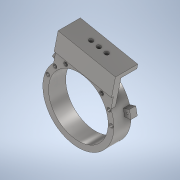
# Autodesk Inventor part: 02
Saved by Autodesk Inventor 2021 (Build 250183000, 183)
## iProperties
Created: 2021-01-15
Part Number: 02
Material: Edelstahl
Document SubType Name: Modeling
Designer: Daniel Dux
Density: 8 g/cm^3
Appearance: Halbpoliert
Mass: 1022.9 g
Surface Area: 385.122 cm^2
Volume: 127.862 cm^3
d117: 94,000 mm
d118: 112,000 mm
d119: 104,000 mm
d120: 5,000 mm
d121: 7,000 mm
d122: 94,000 mm
d123: 5,000 mm
d124: 10,000 mm
d125: 112,000 mm
d208: 98,000 mm
d209: 112,000 mm
d210: 104,000 mm
d211: 5,000 mm
d212: 7,000 mm
d213: 98,000 mm
d214: 5,000 mm
d215: 10,000 mm
d216: 112,000 mm
d217: 20,000 mm
d236: 94,000 mm
d237: 112,000 mm
d238: 104,000 mm
d239: 6,000 mm
d240: 7,000 mm
d241: 98,000 mm
d242: 8,000 mm
d243: 10,000 mm
Author: Daniel Dux
Title: Oberer Mount
Autodesk Inventor part; units mm, degrees
sketch "Skizze1" plane through (0, 0, 0) normal (0, 0, 1) x (1, 0, 0)
  circle A0 centre (0, 0) radius 47
  circle A1 centre (0, 0) radius 56
  circle A2 centre (0, 0) radius 51.5
  circle A3 centre (-28.6119, 42.8207) radius 6
  circle A4 centre (-42.8207, 28.6119) radius 6
  circle A5 centre (42.8207, 28.6119) radius 6
  circle A6 centre (50.5104, 10.0472) radius 6
  circle A7 centre (-10.0472, -50.5104) radius 6
  circle A8 centre (-28.6119, 42.8207) radius 5
  circle A9 centre (-42.8207, 28.6119) radius 5
  circle A10 centre (-10.0472, -50.5104) radius 5
  circle A11 centre (50.5104, 10.0472) radius 5
  circle A12 centre (42.8207, 28.6119) radius 5
  line L0 (0, 0) -> (-25.4753, 49.8699)
  line L1 (0, 0) -> (-26.4443, 49.3629)
  line L2 (0, 0) -> (-36.3248, 42.6205)
  line L3 (0, 0) -> (-35.4856, 43.3218)
  line L4 (0, 0) -> (-42.6205, 36.3248)
  line L5 (0, 0) -> (-49.3629, 26.4443)
  line L6 (0, 0) -> (-49.8699, 25.4753)
  line L7 (0, 0) -> (-43.3218, 35.4856)
  line L8 (0, 0) -> (-16.2059, -53.6038)
  line L9 (0, 0) -> (-17.2496, -53.2771)
  line L10 (0, 0) -> (-5.541, -55.7252)
  line L11 (0, 0) -> (-4.4517, -55.8228)
  line L12 (0, 0) -> (43.3218, 35.4856)
  line L13 (0, 0) -> (42.6205, 36.3248)
  line L14 (0, 0) -> (49.3629, 26.4443)
  line L15 (0, 0) -> (49.8699, 25.4753)
  line L16 (0, 0) -> (53.6038, 16.2059)
  line L17 (0, 0) -> (53.2771, 17.2496)
  line L18 (0, 0) -> (55.7252, 5.541)
  line L19 (0, 0) -> (55.8228, 4.4517)
  line L20 (0, 0) -> (-54.924, 10.9251)
  line L21 (0, 0) -> (54.924, -10.9251)
  line L22 (0, 0) -> (10.0472, 50.5104)
  point P0 (0, 51.5)
  point P1 (-10.0472, 50.5104)
  point P2 (-19.7082, 47.5798)
  point P3 (-36.416, 36.416)
  point P4 (-47.5798, 19.7082)
  point P5 (-50.5104, 10.0472)
  point P6 (-51.5, 0)
  point P7 (-50.5104, -10.0472)
  point P8 (-47.5798, -19.7082)
  point P9 (-42.8207, -28.6119)
  point P10 (-36.416, -36.416)
  point P11 (-28.6119, -42.8207)
  point P12 (-19.7082, -47.5798)
  point P13 (0, -51.5)
  point P14 (10.0472, -50.5104)
  point P15 (19.7082, -47.5798)
  point P16 (28.6119, -42.8207)
  point P17 (36.416, -36.416)
  point P18 (42.8207, -28.6119)
  point P19 (47.5798, -19.7082)
  point P20 (50.5104, -10.0472)
  point P21 (51.5, 0)
  point P22 (47.5798, 19.7082)
  point P23 (36.416, 36.416)
  point P24 (28.6119, 42.8207)
  point P25 (19.7082, 47.5798)
  point P26 (-41.8551, 21.3811)
  point P27 (-41.4296, 22.1944)
  point P28 (-36.3593, 29.7825)
  point P29 (-35.7708, 30.4869)
  point P30 (-30.3782, 37.0866)
  point P31 (-30.4869, 35.7708)
  point P32 (-29.1766, 36.8473)
  point P33 (-22.6383, 42.2582)
  point P34 (-22.8771, 41.0565)
  point P35 (-21.3811, 41.8551)
  point P36 (-14.4773, -44.7147)
  point P37 (-13.6014, -44.9889)
  point P38 (-3.7363, -46.8513)
  point P39 (-4.6505, -46.7694)
  point P40 (46.7694, 4.6505)
  point P41 (46.8513, 3.7363)
  point P42 (44.7147, 14.4773)
  point P43 (44.9889, 13.6014)
  point P44 (41.4296, 22.1944)
  point P45 (41.8551, 21.3811)
  point P46 (35.7708, 30.4869)
  point P47 (36.3593, 29.7825)
  dimension "d1" = 112
  dimension "d2" = 103
  dimension "d0" = 94
  dimension "d5" = 360
  dimension "d7" = 12
  dimension "d8" = 12
  dimension "d9" = 12
  dimension "d10" = 12
  dimension "d11" = 12
  dimension "d12" = 10
  dimension "d13" = 10
  dimension "d14" = 10
  dimension "d15" = 10
  dimension "d16" = 10
  constraints: 12 coincident, 11 centre point, 1 end point, 128 other
  measures "d0" diameter of A0
  measures "d7" diameter of A3
  measures "d8" diameter of A4
  measures "d9" diameter of A5
  measures "d10" diameter of A6
  measures "d11" diameter of A7
  measures "d12" diameter of A8
  measures "d13" diameter of A9
  measures "d14" diameter of A10
  measures "d15" diameter of A11
  measures "d16" diameter of A12
ref_plane "Arbeitsebene1" through (0, 0, 10) normal (0, 0, 1) x (1, 0, 0)
sketch "Skizze2" plane through (0, 0, 10) normal (0, 0, 1) x (1, 0, 0)
  circle A0 centre (0, 0) radius 47
  circle A1 centre (0, 0) radius 56
  arc A2 (-42.7016, 36.2295) -> (-43.3876, 35.405) centre (0, 0) ccw projected
  line L0 (0, 0) -> (-25.5867, 49.8129)
  arc A3 (55.8127, 4.5765) -> (55.7148, 5.6445) centre (0, 0) ccw projected
  line L1 (-22.3883, 43.5863) -> (-25.5867, 49.8129) projected
  circle A4 centre (0, 0) radius 47
  circle A5 centre (0, 0) radius 56
  circle A6 centre (0, 0) radius 52.5
  line L2 (0, 0) -> (-25.5867, 49.8129)
  point P0 (-21.4745, 41.8072)
  point P1 (0, 52.5)
  point P2 (-10.2422, 51.4912)
  point P3 (-20.0909, 48.5037)
  point P4 (-29.1674, 43.6522)
  point P5 (-37.1231, 37.1231)
  point P6 (-43.6522, 29.1674)
  point P7 (-48.5037, 20.0909)
  point P8 (-51.4912, 10.2422)
  point P9 (-52.5, 0)
  point P10 (-51.4912, -10.2422)
  point P11 (-48.5037, -20.0909)
  point P12 (-43.6522, -29.1674)
  point P13 (-37.1231, -37.1231)
  point P14 (-29.1674, -43.6522)
  point P15 (-20.0909, -48.5037)
  point P16 (-10.2422, -51.4912)
  point P17 (0, -52.5)
  point P18 (10.2422, -51.4912)
  point P19 (20.0909, -48.5037)
  point P20 (29.1674, -43.6522)
  point P21 (37.1231, -37.1231)
  point P22 (43.6522, -29.1674)
  point P23 (48.5037, -20.0909)
  point P24 (51.4912, -10.2422)
  point P25 (52.5, 0)
  point P26 (51.4912, 10.2422)
  point P27 (48.5037, 20.0909)
  point P28 (43.6522, 29.1674)
  point P29 (37.1231, 37.1231)
  point P30 (29.1674, 43.6522)
  point P31 (20.0909, 48.5037)
  point P32 (10.2422, 51.4912)
  point P33 (-43.5863, 22.3883)
  point P34 (-43.1495, 23.219)
  point P35 (-37.9642, 30.9794)
  point P36 (-37.3639, 31.7008)
  point P37 (-30.9445, 37.9213)
  point P38 (-31.7008, 37.3639)
  point P39 (-31.0074, 37.9413)
  point P40 (-23.1928, 43.1008)
  point P41 (-23.1871, 43.1666)
  point P42 (-14.9892, -46.6511)
  point P43 (-14.093, -46.9296)
  point P44 (-4.0044, -48.8361)
  point P45 (-4.939, -48.7505)
  point P46 (48.7505, 4.939)
  point P47 (48.8361, 4.0044)
  point P48 (46.6511, 14.9892)
  point P49 (46.9296, 14.093)
  point P50 (43.1495, 23.219)
  point P51 (43.5863, 22.3883)
  point P52 (37.3639, 31.7008)
  point P53 (37.9642, 30.9794)
  dimension "d19" = 94
  dimension "d81" = 112
  dimension "d82" = 105
  dimension "d20" = 112
  dimension "d80" = 94
  dimension "d83" = 360
  constraints: 5 coincident, 4 end point, 2 centre point, 1 collinear, 1 vertical alignment, 40 other
  measures "d20" diameter of A1
  measures "d80" diameter of A4
extrude "Extrusion2" add sketch "Skizze2" along normal blind 10 contours A1 | A6
ref_plane "Arbeitsebene2" through (0, 0, 20) normal (0, 0, 1) x (1, 0, 0)
sketch "Skizze3" plane through (0, 0, 20) normal (0, 0, 1) x (1, 0, 0)
  circle A0 centre (0, 0) radius 47
  circle A1 centre (0, 0) radius 56
  dimension "d30" = 94
  dimension "d31" = 112
  constraints: 2 centre point, 2 coincident
  measures "d30" diameter of A0
  measures "d31" diameter of A1
extrude "Extrusion3" add sketch "Skizze3" along normal blind 10
ref_plane "Arbeitsebene3" through (0, 0, 30) normal (0, 0, 1) x (1, 0, 0)
sketch "Skizze4" plane through (0, 0, 30) normal (0, 0, 1) x (1, 0, 0)
  circle A0 centre (0, 0) radius 49 projected
  line L0 (-22.188, 43.8818) -> (37.2918, 32.0506)
  line L1 (37.2918, 32.0506) -> (44.6056, 68.8203)
  line L2 (44.6056, 68.8203) -> (-14.8741, 80.6514)
  line L3 (-14.8741, 80.6514) -> (-22.188, 43.8818)
  line L4 (44.6056, 68.8203) -> (37.2918, 32.0506)
  line L5 (37.2918, 32.0506) -> (52.7171, 28.9824)
  line L6 (48.4587, 7.5737) -> (60.031, 65.752)
  line L7 (60.031, 65.752) -> (44.6056, 68.8203)
  line L8 (-14.8741, 80.6514) -> (-22.188, 43.8818)
  line L9 (-22.188, 43.8818) -> (-37.6133, 46.9501)
  line L10 (-41.8717, 25.5414) -> (-30.2994, 83.7197)
  line L11 (-30.2994, 83.7197) -> (-14.8741, 80.6514)
  circle A1 centre (0, 0) radius 56
  circle A2 centre (0, 0) radius 47
  point P0 (-38.9486, 40.2369)
  point P1 (51.3817, 22.2692)
  point P2 (-22.174, 43.6957)
  point P3 (37.2076, 31.884)
  point P4 (-41.8227, 25.5317)
  point P5 (48.4096, 7.5835)
  point P6 (37.0169, 32.1053)
  point P7 (-21.9131, 43.8271)
  dimension "AuslegerBreite" = 92.1
  dimension "d34" = 37.49
  dimension "d37" = 15.7275
  dimension "d38" = 15.7275
  dimension "d39" = 92.1
  dimension "d40" = 60.645
  dimension "d55" = 112
  dimension "d136" = 98
  dimension "d137" = 94
  dimension "d138" = 76.2
  constraints: 24 end point, 6 parallel, 4 perpendicular, 2 centre point, 2 coincident, 2 point on line
  measures "d34" distance of L0.end L1.end
  measures "d37" distance between parallel lines of L1 L6
  measures "d38" distance between parallel lines of L10 L3
  measures "d39" distance between parallel lines of L10 L6
  measures "d40" distance between parallel lines of L3 L1
  measures "d55" diameter of A1
  measures "d136" diameter of A0
  measures "d137" diameter of A2
  measures "d138" distance from line of point (0, 0) L2
extrude "Extrusion4" add sketch "Skizze4" along normal blind 7 contours A0 L0 A2 | A0 L0 L5 A1 L9 | L0 A2 A0 | A0 L0 L3 A1 L1 | L1 A1 L5 | L9 A1 L3 | A1 L3 L2 L1 | L1 L7 L6 L5 A1 | L5 L6 A1 | A1 L9 L10 L11 L3 | A1 L10 L9
ref_plane "Arbeitsebene4" through (0, 0, 45) normal (0, 0, 1) x (1, 0, 0)
sketch "Skizze7" plane through (0, 0, 10) normal (0, 0, 1) x (1, 0, 0)
  circle A0 centre (0, 0) radius 47
  circle A1 centre (0, 0) radius 56
  circle A2 centre (0, 0) radius 52.5
  circle A3 centre (-29.1674, 43.6522) radius 6
  circle A4 centre (-43.6522, 29.1674) radius 6
  circle A5 centre (43.6522, 29.1674) radius 6
  circle A6 centre (51.4912, 10.2422) radius 6
  circle A7 centre (-10.2422, -51.4912) radius 6
  circle A8 centre (-29.1674, 43.6522) radius 5
  circle A9 centre (-43.6522, 29.1674) radius 5
  circle A10 centre (-10.2422, -51.4912) radius 5
  circle A11 centre (51.4912, 10.2422) radius 5
  circle A12 centre (43.6522, 29.1674) radius 5
  line L0 (0, 0) -> (-25.5867, 49.8129)
  line L1 (0, 0) -> (-26.536, 49.3137)
  line L2 (0, 0) -> (-36.2295, 42.7016)
  line L3 (0, 0) -> (-35.405, 43.3876)
  line L4 (0, 0) -> (-42.7016, 36.2295)
  line L5 (0, 0) -> (-49.3137, 26.536)
  line L6 (0, 0) -> (-49.8129, 25.5867)
  line L7 (0, 0) -> (-43.3876, 35.405)
  line L8 (0, 0) -> (-16.1063, -53.6338)
  line L9 (0, 0) -> (-17.1305, -53.3155)
  line L10 (0, 0) -> (-5.6445, -55.7148)
  line L11 (0, 0) -> (-4.5765, -55.8127)
  line L12 (0, 0) -> (43.3876, 35.405)
  line L13 (0, 0) -> (42.7016, 36.2295)
  line L14 (0, 0) -> (49.3137, 26.536)
  line L15 (0, 0) -> (49.8129, 25.5867)
  line L16 (0, 0) -> (53.6338, 16.1063)
  line L17 (0, 0) -> (53.3155, 17.1305)
  line L18 (0, 0) -> (55.7148, 5.6445)
  line L19 (0, 0) -> (55.8127, 4.5765)
  line L20 (0, 0) -> (-54.924, 10.9251)
  line L21 (0, 0) -> (54.924, -10.9251)
  point P0 (0, 52.5)
  point P1 (-10.2422, 51.4912)
  point P2 (-20.0909, 48.5037)
  point P3 (-37.1231, 37.1231)
  point P4 (-48.5037, 20.0909)
  point P5 (-51.4912, 10.2422)
  point P6 (-52.5, 0)
  point P7 (-51.4912, -10.2422)
  point P8 (-48.5037, -20.0909)
  point P9 (-43.6522, -29.1674)
  point P10 (-37.1231, -37.1231)
  point P11 (-29.1674, -43.6522)
  point P12 (-20.0909, -48.5037)
  point P13 (0, -52.5)
  point P14 (10.2422, -51.4912)
  point P15 (20.0909, -48.5037)
  point P16 (29.1674, -43.6522)
  point P17 (37.1231, -37.1231)
  point P18 (43.6522, -29.1674)
  point P19 (48.5037, -20.0909)
  point P20 (51.4912, -10.2422)
  point P21 (52.5, 0)
  point P22 (48.5037, 20.0909)
  point P23 (37.1231, 37.1231)
  point P24 (29.1674, 43.6522)
  point P25 (20.0909, 48.5037)
  point P26 (10.2422, 51.4912)
  point P27 (-43.5863, 22.3883)
  point P28 (-43.1495, 23.219)
  point P29 (-37.9642, 30.9794)
  point P30 (-37.3639, 31.7008)
  point P31 (-30.9445, 37.9213)
  point P32 (-31.7008, 37.3639)
  point P33 (-31.0074, 37.9413)
  point P34 (-23.1928, 43.1008)
  point P35 (-23.1871, 43.1666)
  point P36 (-22.3883, 43.5863)
  point P37 (-14.9892, -46.6511)
  point P38 (-14.093, -46.9296)
  point P39 (-4.0044, -48.8361)
  point P40 (-4.939, -48.7505)
  point P41 (48.7505, 4.939)
  point P42 (48.8361, 4.0044)
  point P43 (46.6511, 14.9892)
  point P44 (46.9296, 14.093)
  point P45 (43.1495, 23.219)
  point P46 (43.5863, 22.3883)
  point P47 (37.3639, 31.7008)
  point P48 (37.9642, 30.9794)
  point P49 (51.4912, -10.2422)
  point P50 (52.3244, 4.2904)
  point P51 (-51.4912, 10.2422)
  point P52 (-46.0969, 9.1692)
  point P53 (-41.8072, 21.4745)
  point P54 (-46.6996, 23.9875)
  point P55 (46.0969, -9.1692)
  point P56 (46.8428, 3.8409)
  dimension "d59" = 112
  dimension "d60" = 105
  dimension "d58" = 94
  dimension "d61" = 360
  dimension "d62" = 12
  dimension "d63" = 12
  dimension "d64" = 12
  dimension "d65" = 12
  dimension "d66" = 12
  dimension "d67" = 10
  dimension "d68" = 10
  dimension "d69" = 10
  dimension "d70" = 10
  dimension "d71" = 10
  constraints: 44 end point, 20 tangent, 13 coincident, 11 centre point, 2 point on line, 60 other
  measures "d58" diameter of A0
  measures "d62" diameter of A3
  measures "d63" diameter of A4
  measures "d64" diameter of A5
  measures "d65" diameter of A6
  measures "d66" diameter of A7
  measures "d67" diameter of A8
  measures "d68" diameter of A9
  measures "d69" diameter of A10
  measures "d70" diameter of A11
  measures "d71" diameter of A12
sketch "Skizze8" plane through (0, 0, 10) normal (0, 0, -1) x (-1, 0, 0)
  circle A0 centre (0, 0) radius 47
  circle A1 centre (0, 0) radius 56
  circle A2 centre (0, 0) radius 52
  circle A3 centre (0, 52) radius 2.5
  circle A4 centre (-19.8995, 48.0417) radius 2.5
  circle A5 centre (-36.7696, 36.7696) radius 2.5
  circle A6 centre (-48.0417, 19.8995) radius 2.5
  circle A7 centre (-52, 0) radius 2.5
  circle A8 centre (-48.0417, -19.8995) radius 2.5
  circle A9 centre (-36.7696, -36.7696) radius 2.5
  circle A10 centre (-19.8995, -48.0417) radius 2.5
  circle A11 centre (0, -52) radius 2.5
  circle A12 centre (19.8995, -48.0417) radius 2.5
  circle A13 centre (36.7696, -36.7696) radius 2.5
  circle A14 centre (48.0417, -19.8995) radius 2.5
  circle A15 centre (52, 0) radius 2.5
  circle A16 centre (48.0417, 19.8995) radius 2.5
  circle A17 centre (36.7696, 36.7696) radius 2.5
  circle A18 centre (19.8995, 48.0417) radius 2.5
  circle A19 centre (0, -52) radius 3.5
  circle A20 centre (19.8995, -48.0417) radius 3.5
  line L0 (0, 0) -> (-3.7692, -55.873)
  line L1 (0, 0) -> (24.864, -50.1775)
  line L2 (-54.924, -10.9251) -> (-48.0585, -9.5594)
  line L3 (0, 0) -> (-54.924, -10.9251)
  line L4 (48.0585, 9.5594) -> (54.924, 10.9251)
  line L5 (0, 0) -> (54.924, 10.9251)
  circle A21 centre (0, 0) radius 47
  line L6 (-27.2229, 40.742) -> (-31.1119, 46.5623)
  line L7 (0, 0) -> (-31.1119, 46.5623)
  line L8 (10.9251, 54.924) -> (9.5594, 48.0585)
  line L9 (0, 0) -> (10.9251, 54.924)
  circle A22 centre (0, 52) radius 2.5
  circle A23 centre (-10.1447, 51.0008) radius 2.5
  circle A24 centre (-19.8995, 48.0417) radius 2.5
  circle A25 centre (-28.8897, 43.2364) radius 2.5
  circle A26 centre (-36.7696, 36.7696) radius 2.5
  circle A27 centre (-43.2364, 28.8897) radius 2.5
  circle A28 centre (-48.0417, 19.8995) radius 2.5
  circle A29 centre (-51.0008, 10.1447) radius 2.5
  circle A30 centre (-52, 0) radius 2.5
  circle A31 centre (-51.0008, -10.1447) radius 2.5
  circle A32 centre (-48.0417, -19.8995) radius 2.5
  circle A33 centre (-43.2364, -28.8897) radius 2.5
  circle A34 centre (-36.7696, -36.7696) radius 2.5
  circle A35 centre (-28.8897, -43.2364) radius 2.5
  circle A36 centre (-19.8995, -48.0417) radius 2.5
  circle A37 centre (-10.1447, -51.0008) radius 2.5
  circle A38 centre (0, -52) radius 2.5
  circle A39 centre (10.1447, -51.0008) radius 2.5
  circle A40 centre (19.8995, -48.0417) radius 2.5
  circle A41 centre (28.8897, -43.2364) radius 2.5
  circle A42 centre (36.7696, -36.7696) radius 2.5
  circle A43 centre (43.2364, -28.8897) radius 2.5
  circle A44 centre (48.0417, -19.8995) radius 2.5
  circle A45 centre (51.0008, -10.1447) radius 2.5
  circle A46 centre (52, 0) radius 2.5
  circle A47 centre (51.0008, 10.1447) radius 2.5
  circle A48 centre (48.0417, 19.8995) radius 2.5
  circle A49 centre (43.2364, 28.8897) radius 2.5
  circle A50 centre (36.7696, 36.7696) radius 2.5
  circle A51 centre (28.8897, 43.2364) radius 2.5
  circle A52 centre (19.8995, 48.0417) radius 2.5
  circle A53 centre (10.1447, 51.0008) radius 2.5
  circle A54 centre (28.8897, 43.2364) radius 5 construction
  line L10 (0, 0) -> (26.4906, 49.3381)
  arc A55 (54.924, 10.9251) -> (10.9251, 54.924) centre (0, 0) ccw
  line L11 (0, 0) -> (35.4449, 43.355)
  line L12 (0, 0) -> (5.5933, 55.72)
  line L13 (0, 0) -> (16.1556, 53.619)
  line L14 (0, 0) -> (-16.1556, 53.619)
  line L15 (0, 0) -> (-5.5933, 55.72)
  line L16 (0, 0) -> (-35.4449, 43.355)
  line L17 (0, 0) -> (-26.4906, 49.3381)
  line L18 (0, 0) -> (-49.3381, 26.4906)
  line L19 (0, 0) -> (-43.355, 35.4449)
  line L20 (0, 0) -> (-55.72, 5.5933)
  line L21 (0, 0) -> (-53.619, 16.1556)
  line L22 (0, 0) -> (-53.619, -16.1556)
  line L23 (0, 0) -> (-55.72, -5.5933)
  line L24 (0, 0) -> (-43.355, -35.4449)
  line L25 (0, 0) -> (-49.3381, -26.4906)
  line L26 (0, 0) -> (-26.4906, -49.3381)
  line L27 (0, 0) -> (-35.4449, -43.355)
  line L28 (0, 0) -> (-5.5933, -55.72)
  line L29 (0, 0) -> (-16.1556, -53.619)
  line L30 (0, 0) -> (16.1556, -53.619)
  line L31 (0, 0) -> (5.5933, -55.72)
  line L32 (0, 0) -> (35.4449, -43.355)
  line L33 (0, 0) -> (26.4906, -49.3381)
  line L34 (0, 0) -> (49.3381, -26.4906)
  line L35 (0, 0) -> (43.355, -35.4449)
  line L36 (0, 0) -> (55.72, -5.5933)
  line L37 (0, 0) -> (53.619, -16.1556)
  line L38 (0, 0) -> (53.619, 16.1556)
  line L39 (0, 0) -> (55.72, 5.5933)
  line L40 (0, 0) -> (43.355, 35.4449)
  line L41 (0, 0) -> (49.3381, 26.4906)
  circle A56 centre (0, 0) radius 66
  line L42 (0, 0) -> (51.097, 41.7744)
  line L43 (0, 0) -> (58.1485, 31.2211)
  line L44 (0, 0) -> (6.5921, -65.67)
  line L45 (0, 0) -> (19.0405, -63.1938)
  line L46 (0, 0) -> (-63.1938, 19.0405)
  line L47 (0, 0) -> (-65.67, 6.5921)
  line L48 (0, 0) -> (-59.8279, 11.9005)
  line L49 (0, 0) -> (50.7196, 33.8898)
  line L50 (0, 0) -> (11.9005, -59.8279)
  circle A57 centre (0, 0) radius 49
  circle A58 centre (0, 0) radius 56
  circle A59 centre (0, 0) radius 52
  circle A60 centre (0, 52) radius 2.5
  circle A61 centre (-19.8995, 48.0417) radius 2.5
  circle A62 centre (-36.7696, 36.7696) radius 2.5
  circle A63 centre (-48.0417, 19.8995) radius 2.5
  circle A64 centre (-52, 0) radius 2.5
  circle A65 centre (-48.0417, -19.8995) radius 2.5
  circle A66 centre (-36.7696, -36.7696) radius 2.5
  circle A67 centre (-19.8995, -48.0417) radius 2.5
  circle A68 centre (0, -52) radius 2.5
  circle A69 centre (19.8995, -48.0417) radius 2.5
  circle A70 centre (36.7696, -36.7696) radius 2.5
  circle A71 centre (48.0417, -19.8995) radius 2.5
  circle A72 centre (52, 0) radius 2.5
  circle A73 centre (48.0417, 19.8995) radius 2.5
  circle A74 centre (36.7696, 36.7696) radius 2.5
  circle A75 centre (19.8995, 48.0417) radius 2.5
  circle A76 centre (0, -52) radius 3.5
  circle A77 centre (19.8995, -48.0417) radius 3.5
  line L51 (0, 0) -> (-3.7692, -55.873)
  line L52 (0, 0) -> (24.864, -50.1775)
  line L53 (-54.924, -10.9251) -> (-48.0585, -9.5594)
  line L54 (0, 0) -> (-54.924, -10.9251)
  line L55 (48.0585, 9.5594) -> (54.924, 10.9251)
  line L56 (0, 0) -> (54.924, 10.9251)
  circle A78 centre (0, 0) radius 49
  line L57 (-27.2229, 40.742) -> (-31.1119, 46.5623)
  line L58 (0, 0) -> (-31.1119, 46.5623)
  line L59 (10.9251, 54.924) -> (9.5594, 48.0585)
  line L60 (0, 0) -> (10.9251, 54.924)
  circle A79 centre (0, 52) radius 2.5
  circle A80 centre (-10.1447, 51.0008) radius 2.5
  circle A81 centre (-19.8995, 48.0417) radius 2.5
  circle A82 centre (-28.8897, 43.2364) radius 2.5
  circle A83 centre (-36.7696, 36.7696) radius 2.5
  circle A84 centre (-43.2364, 28.8897) radius 2.5
  circle A85 centre (-48.0417, 19.8995) radius 2.5
  circle A86 centre (-51.0008, 10.1447) radius 2.5
  circle A87 centre (-52, 0) radius 2.5
  circle A88 centre (-51.0008, -10.1447) radius 2.5
  circle A89 centre (-48.0417, -19.8995) radius 2.5
  circle A90 centre (-43.2364, -28.8897) radius 2.5
  circle A91 centre (-36.7696, -36.7696) radius 2.5
  circle A92 centre (-28.8897, -43.2364) radius 2.5
  circle A93 centre (-19.8995, -48.0417) radius 2.5
  circle A94 centre (-10.1447, -51.0008) radius 2.5
  circle A95 centre (0, -52) radius 2.5
  circle A96 centre (10.1447, -51.0008) radius 2.5
  circle A97 centre (19.8995, -48.0417) radius 2.5
  circle A98 centre (28.8897, -43.2364) radius 2.5
  circle A99 centre (36.7696, -36.7696) radius 2.5
  circle A100 centre (43.2364, -28.8897) radius 2.5
  circle A101 centre (48.0417, -19.8995) radius 2.5
  circle A102 centre (51.0008, -10.1447) radius 2.5
  circle A103 centre (52, 0) radius 2.5
  circle A104 centre (51.0008, 10.1447) radius 2.5
  circle A105 centre (48.0417, 19.8995) radius 2.5
  circle A106 centre (43.2364, 28.8897) radius 2.5
  circle A107 centre (36.7696, 36.7696) radius 2.5
  circle A108 centre (28.8897, 43.2364) radius 2.5
  circle A109 centre (19.8995, 48.0417) radius 2.5
  circle A110 centre (10.1447, 51.0008) radius 2.5
  circle A111 centre (28.8897, 43.2364) radius 5 construction
  line L61 (0, 0) -> (26.4906, 49.3381)
  arc A112 (54.924, 10.9251) -> (10.9251, 54.924) centre (0, 0) ccw
  line L62 (0, 0) -> (35.4449, 43.355)
  line L63 (0, 0) -> (5.5933, 55.72)
  line L64 (0, 0) -> (16.1556, 53.619)
  line L65 (0, 0) -> (-16.1556, 53.619)
  line L66 (0, 0) -> (-5.5933, 55.72)
  line L67 (0, 0) -> (-35.4449, 43.355)
  line L68 (0, 0) -> (-26.4906, 49.3381)
  line L69 (0, 0) -> (-49.3381, 26.4906)
  line L70 (0, 0) -> (-43.355, 35.4449)
  line L71 (0, 0) -> (-55.72, 5.5933)
  line L72 (0, 0) -> (-53.619, 16.1556)
  line L73 (0, 0) -> (-53.619, -16.1556)
  line L74 (0, 0) -> (-55.72, -5.5933)
  line L75 (0, 0) -> (-43.355, -35.4449)
  line L76 (0, 0) -> (-49.3381, -26.4906)
  line L77 (0, 0) -> (-26.4906, -49.3381)
  line L78 (0, 0) -> (-35.4449, -43.355)
  line L79 (0, 0) -> (-5.5933, -55.72)
  line L80 (0, 0) -> (-16.1556, -53.619)
  line L81 (0, 0) -> (16.1556, -53.619)
  line L82 (0, 0) -> (5.5933, -55.72)
  line L83 (0, 0) -> (35.4449, -43.355)
  line L84 (0, 0) -> (26.4906, -49.3381)
  line L85 (0, 0) -> (49.3381, -26.4906)
  line L86 (0, 0) -> (43.355, -35.4449)
  line L87 (0, 0) -> (55.72, -5.5933)
  line L88 (0, 0) -> (53.619, -16.1556)
  line L89 (0, 0) -> (53.619, 16.1556)
  line L90 (0, 0) -> (55.72, 5.5933)
  line L91 (0, 0) -> (43.355, 35.4449)
  line L92 (0, 0) -> (49.3381, 26.4906)
  circle A113 centre (0, 0) radius 66
  line L93 (0, 0) -> (51.097, 41.7744)
  line L94 (0, 0) -> (58.1485, 31.2211)
  line L95 (0, 0) -> (6.5921, -65.67)
  line L96 (0, 0) -> (19.0405, -63.1938)
  line L97 (0, 0) -> (-63.1938, 19.0405)
  line L98 (0, 0) -> (-65.67, 6.5921)
  circle A114 centre (0, 0) radius 61
  line L99 (0, 0) -> (-59.8279, 11.9005)
  line L100 (0, 0) -> (50.7196, 33.8898)
  line L101 (0, 0) -> (11.9005, -59.8279)
  line L102 (0, 0) -> (-41.7744, -51.097)
  line L103 (0, 0) -> (-31.2211, -58.1485)
  line L104 (0, 0) -> (-33.8898, -50.7196)
  line L105 (-31.1119, -46.5623) -> (-26.1118, -39.0791)
  line L106 (0, 0) -> (51.097, -41.7744)
  line L107 (0, 0) -> (58.1485, -31.2211)
  line L108 (0, 0) -> (50.7196, -33.8898)
  point P0 (21.756, -43.9053)
  point P1 (-3.2981, -48.8889)
  point P2 (-48.755, 4.8941)
  point P3 (-46.9166, 14.1361)
  point P4 (-43.1708, 23.1793)
  point P5 (-37.9356, 31.0143)
  point P6 (14.1361, -46.9166)
  point P7 (4.8941, -48.755)
  point P8 (37.9356, 31.0143)
  point P9 (43.1708, 23.1793)
  point P10 (23.1793, 43.1708)
  point P11 (31.0143, 37.9356)
  point P12 (45.2701, 18.7515)
  point P13 (34.6482, 34.6482)
  point P14 (18.7515, 45.2701)
  point P15 (-34.6482, 34.6482)
  point P16 (-18.7515, 45.2701)
  point P17 (0, 49)
  point P18 (-45.2701, 18.7515)
  point P19 (-49, 0)
  dimension "d104" = 94
  dimension "d106" = 104
  dimension "d195" = 112
  dimension "d196" = 104
  dimension "d206" = 132
  dimension "d105" = 112
  dimension "d107" = 5
  dimension "d108" = 360
  dimension "d109" = 7
  dimension "d110" = 7
  dimension "d111" = 94
  dimension "d112" = 5
  dimension "d113" = 360
  dimension "d114" = 10
  dimension "d115" = 360
  dimension "d116" = 132
  dimension "d194" = 98
  dimension "d197" = 5
  dimension "d198" = 360
  dimension "d199" = 7
  dimension "d200" = 7
  dimension "d201" = 98
  dimension "d202" = 5
  dimension "d203" = 360
  dimension "d204" = 10
  dimension "d205" = 360
  dimension "d207" = 122
  constraints: 218 end point, 110 centre point, 25 collinear, 23 coincident, 21 point on circle, 8 point on line, 8 tangent, 2 vertical alignment, 408 other
  measures "d105" diameter of A1
  measures "d107" diameter of A3
  measures "d109" diameter of A19
  measures "d110" diameter of A20
  measures "d111" diameter of A21
  measures "d112" diameter of A22
  measures "d114" diameter of A54
  measures "d116" diameter of A56
  measures "d194" diameter of A57
  measures "d197" diameter of A60
  measures "d199" diameter of A76
  measures "d200" diameter of A77
  measures "d201" diameter of A78
  measures "d202" diameter of A79
  measures "d204" diameter of A111
  measures "d207" diameter of A114
extrude "Extrusion6" add sketch "Skizze8" against normal blind 10 contours L47 A114 L48 A1 | A1 L48 A114 L46 | L107 A114 L108 A1 | A1 L108 A114 L106 | L42 A114 L49 A1 | A1 L49 A114 L43 | L47 A56 L46 A114 | L107 A56 L106 A114 | L42 A56 L43 A114
hole "Bohrung3" at (59.8279, 11.9005, 10) at (-50.7196, 33.8898, 10) at (-50.7196, -33.8898, 10) direction (0, 0, 1) diameter 3.2 end through all
sketch "Skizze9" plane through (-30.2994, 83.7197, 37) normal (0.1950891, 0.9807855, 0) x (0.9807855, -0.1950891, 0)
  line L0 (0, 7) -> (92.1, 7) projected
  line L1 (92.1, 7) -> (0, 7)
  line L2 (0, 7) -> (0, -18.1)
  line L3 (0, -18.1) -> (92.1, -18.1)
  line L4 (92.1, -18.1) -> (92.1, 7)
  line L5 (92.1, 0) -> (0, 0) projected
  line L6 (92.1, 0) -> (0, 0)
  line L7 (0, 0) -> (0, 32.1)
  line L8 (0, 32.1) -> (92.1, 32.1)
  line L9 (92.1, 32.1) -> (92.1, 0)
  line L10 (0, 7) -> (0, 0) projected
  line L11 (92.1, 0) -> (0, 0)
  line L12 (0, 0) -> (0, -3)
  line L13 (0, -3) -> (92.1, -3)
  line L14 (92.1, -3) -> (92.1, 0)
  point P0 (46.05, 37)
  point P1 (0, -3)
  point P2 (92.1, -3)
  dimension "d139" = 25.1
  dimension "d145" = 32.1
  dimension "d146" = 3
  constraints: 24 end point, 8 equal length, 4 perpendicular
  measures "d139" distance of L2.end L0.start
  measures "d145" distance of L5.end L7.end
  measures "d146" distance of L12.end L5.end
extrude "Extrusion7" add sketch "Skizze9" along normal blind 7 contours L7 L8 L9 L0 | L0 L4 L5 L2 | L5 L4 L13 L2
sketch "Skizze10" plane through (0, 0, 37) normal (0, 0, 1) x (1, 0, 0)
  line L0 (51.3817, 22.2692) -> (60.031, 65.752) projected
  line L1 (-30.2994, 83.7197) -> (-38.9486, 40.2369) projected
  line L2 (60.031, 65.752) -> (-30.2994, 83.7197)
  line L3 (-30.2994, 83.7197) -> (-35.1766, 59.2001)
  line L4 (-35.1766, 59.2001) -> (55.1537, 41.2324)
  line L5 (55.1537, 41.2324) -> (60.031, 65.752)
  point P0 (0, 0)
  dimension "d142" = 25
  constraints: 8 end point, 2 parallel, 2 perpendicular
  measures "d142" distance of L3.end L1.start
extrude "Extrusion8" add sketch "Skizze10" along normal blind 3
sketch "Skizze12" plane through (-28.9338, 90.5852, 37) normal (0.1950891, 0.9807855, 0) x (0.9807855, -0.1950891, 0)
  line L0 (92.1, -3) -> (92.1, 32.1) projected
  line L1 (0, -3) -> (92.1, -3) projected
  line L2 (92.1, -3) -> (0, -3)
  line L3 (0, -3) -> (0, 16)
  line L4 (0, 16) -> (92.1, 16)
  line L5 (92.1, 16) -> (92.1, -3)
  point P0 (46.05, 37)
  point P1 (46.05, 16)
  point P2 (33.55, 16)
  point P3 (58.55, 16)
  dimension "d147" = 19
  dimension "d148" = 92.1
  dimension "d149" = 46.05
  dimension "d150" = 12.5
  dimension "d151" = 12.5
  constraints: 8 end point, 2 parallel, 2 point on line, 1 horizontal, 1 midpoint, 1 perpendicular
  measures "d147" distance of L1.start L3.end
  measures "d148" distance of L3.end L4.end
  measures "d149" distance of L4.end point (46.05, 16)
  measures "d150" distance of point (33.55, 16) point (46.05, 16)
  measures "d151" distance of point (58.55, 16) point (46.05, 16)
hole "Bohrung4" at (16.2314, 81.6014, 21) at (3.9716, 84.04, 21) at (28.4912, 79.1627, 21) direction (-0.1950891, -0.9807855, 0) diameter 6.6 depth 15
sketch "Skizze13" plane through (0, 0, 10) normal (0, 0, 1) x (1, 0, 0)
  circle A0 centre (0, 0) radius 47
  circle A1 centre (0, 0) radius 56
  circle A2 centre (0, 0) radius 51.5
  circle A3 centre (-28.6119, 42.8207) radius 6
  circle A4 centre (-42.8207, 28.6119) radius 6
  circle A5 centre (42.8207, 28.6119) radius 6
  circle A6 centre (50.5104, 10.0472) radius 6
  circle A7 centre (-10.0472, -50.5104) radius 6
  circle A8 centre (-28.6119, 42.8207) radius 5
  circle A9 centre (-42.8207, 28.6119) radius 5
  circle A10 centre (-10.0472, -50.5104) radius 5
  circle A11 centre (50.5104, 10.0472) radius 5
  circle A12 centre (42.8207, 28.6119) radius 5
  line L0 (0, 0) -> (-25.4753, 49.8699)
  line L1 (0, 0) -> (-26.4443, 49.3629)
  line L2 (0, 0) -> (-36.3248, 42.6205)
  line L3 (0, 0) -> (-35.4856, 43.3218)
  line L4 (0, 0) -> (-42.6205, 36.3248)
  line L5 (0, 0) -> (-49.3629, 26.4443)
  line L6 (0, 0) -> (-49.8699, 25.4753)
  line L7 (0, 0) -> (-43.3218, 35.4856)
  line L8 (0, 0) -> (-16.2059, -53.6038)
  line L9 (0, 0) -> (-17.2496, -53.2771)
  line L10 (0, 0) -> (-5.541, -55.7252)
  line L11 (0, 0) -> (-4.4517, -55.8228)
  line L12 (0, 0) -> (43.3218, 35.4856)
  line L13 (0, 0) -> (42.6205, 36.3248)
  line L14 (0, 0) -> (49.3629, 26.4443)
  line L15 (0, 0) -> (49.8699, 25.4753)
  line L16 (0, 0) -> (53.6038, 16.2059)
  line L17 (0, 0) -> (53.2771, 17.2496)
  line L18 (0, 0) -> (55.7252, 5.541)
  line L19 (0, 0) -> (55.8228, 4.4517)
  line L20 (0, 0) -> (-54.924, 10.9251)
  line L21 (0, 0) -> (54.924, -10.9251)
  line L22 (0, 0) -> (10.0472, 50.5104)
  point P0 (0, 51.5)
  point P1 (-10.0472, 50.5104)
  point P2 (-19.7082, 47.5798)
  point P3 (-36.416, 36.416)
  point P4 (-47.5798, 19.7082)
  point P5 (-50.5104, 10.0472)
  point P6 (-51.5, 0)
  point P7 (-50.5104, -10.0472)
  point P8 (-47.5798, -19.7082)
  point P9 (-42.8207, -28.6119)
  point P10 (-36.416, -36.416)
  point P11 (-28.6119, -42.8207)
  point P12 (-19.7082, -47.5798)
  point P13 (0, -51.5)
  point P14 (10.0472, -50.5104)
  point P15 (19.7082, -47.5798)
  point P16 (28.6119, -42.8207)
  point P17 (36.416, -36.416)
  point P18 (42.8207, -28.6119)
  point P19 (47.5798, -19.7082)
  point P20 (50.5104, -10.0472)
  point P21 (51.5, 0)
  point P22 (47.5798, 19.7082)
  point P23 (36.416, 36.416)
  point P24 (28.6119, 42.8207)
  point P25 (19.7082, 47.5798)
  point P26 (-41.8551, 21.3811)
  point P27 (-41.4296, 22.1944)
  point P28 (-36.3593, 29.7825)
  point P29 (-35.7708, 30.4869)
  point P30 (-30.3782, 37.0866)
  point P31 (-30.4869, 35.7708)
  point P32 (-29.1766, 36.8473)
  point P33 (-22.6383, 42.2582)
  point P34 (-22.8771, 41.0565)
  point P35 (-21.3811, 41.8551)
  point P36 (-14.4773, -44.7147)
  point P37 (-13.6014, -44.9889)
  point P38 (-3.7363, -46.8513)
  point P39 (-4.6505, -46.7694)
  point P40 (46.7694, 4.6505)
  point P41 (46.8513, 3.7363)
  point P42 (44.7147, 14.4773)
  point P43 (44.9889, 13.6014)
  point P44 (41.4296, 22.1944)
  point P45 (41.8551, 21.3811)
  point P46 (35.7708, 30.4869)
  point P47 (36.3593, 29.7825)
  dimension "d164" = 112
  dimension "d165" = 103
  dimension "d163" = 94
  dimension "d166" = 360
  dimension "d167" = 12
  dimension "d168" = 12
  dimension "d169" = 12
  dimension "d170" = 12
  dimension "d171" = 12
  dimension "d172" = 10
  dimension "d173" = 10
  dimension "d174" = 10
  dimension "d175" = 10
  dimension "d176" = 10
  constraints: 21 end point, 20 tangent, 12 coincident, 11 centre point, 88 other
  measures "d163" diameter of A0
  measures "d167" diameter of A3
  measures "d168" diameter of A4
  measures "d169" diameter of A5
  measures "d170" diameter of A6
  measures "d171" diameter of A7
  measures "d172" diameter of A8
  measures "d173" diameter of A9
  measures "d174" diameter of A10
  measures "d175" diameter of A11
  measures "d176" diameter of A12
hole "Bohrung5" at (-42.8207, -28.6119, 10) at (-42.8207, 28.6119, 10) at (-28.6119, 42.8207, 10) at (42.8207, 28.6119, 10) at (50.5104, 10.0472, 10) at (50.5104, -10.0472, 10) direction (0, 0, 1) diameter 3 depth 15
sketch "Skizze14" plane through (0, 0, 10) normal (0, 0, -1) x (-1, 0, 0)
  circle A0 centre (0, 0) radius 47
  circle A1 centre (0, 0) radius 56
  circle A2 centre (0, 0) radius 52
  circle A3 centre (0, 52) radius 3
  circle A4 centre (-19.8995, 48.0417) radius 3
  circle A5 centre (-36.7696, 36.7696) radius 3
  circle A6 centre (-48.0417, 19.8995) radius 3
  circle A7 centre (-52, 0) radius 3
  circle A8 centre (-48.0417, -19.8995) radius 3
  circle A9 centre (-36.7696, -36.7696) radius 3
  circle A10 centre (-19.8995, -48.0417) radius 3
  circle A11 centre (0, -52) radius 3
  circle A12 centre (19.8995, -48.0417) radius 3
  circle A13 centre (36.7696, -36.7696) radius 3
  circle A14 centre (48.0417, -19.8995) radius 3
  circle A15 centre (52, 0) radius 3
  circle A16 centre (48.0417, 19.8995) radius 3
  circle A17 centre (36.7696, 36.7696) radius 3
  circle A18 centre (19.8995, 48.0417) radius 3
  circle A19 centre (0, -52) radius 3.5
  circle A20 centre (19.8995, -48.0417) radius 3.5
  line L0 (0, 0) -> (-3.7692, -55.873)
  line L1 (0, 0) -> (24.864, -50.1775)
  line L2 (-54.924, -10.9251) -> (-46.0969, -9.1692)
  line L3 (0, 0) -> (-54.924, -10.9251)
  line L4 (46.0969, 9.1692) -> (54.924, 10.9251)
  line L5 (0, 0) -> (54.924, 10.9251)
  circle A21 centre (0, 0) radius 49
  line L6 (-26.1118, 39.0791) -> (-31.1119, 46.5623)
  line L7 (0, 0) -> (-31.1119, 46.5623)
  line L8 (10.9251, 54.924) -> (9.1692, 46.0969)
  line L9 (0, 0) -> (10.9251, 54.924)
  circle A22 centre (0, 52) radius 4
  circle A23 centre (-10.1447, 51.0008) radius 4
  circle A24 centre (-19.8995, 48.0417) radius 4
  circle A25 centre (-28.8897, 43.2364) radius 4
  circle A26 centre (-36.7696, 36.7696) radius 4
  circle A27 centre (-43.2364, 28.8897) radius 4
  circle A28 centre (-48.0417, 19.8995) radius 4
  circle A29 centre (-51.0008, 10.1447) radius 4
  circle A30 centre (-52, 0) radius 4
  circle A31 centre (-51.0008, -10.1447) radius 4
  circle A32 centre (-48.0417, -19.8995) radius 4
  circle A33 centre (-43.2364, -28.8897) radius 4
  circle A34 centre (-36.7696, -36.7696) radius 4
  circle A35 centre (-28.8897, -43.2364) radius 4
  circle A36 centre (-19.8995, -48.0417) radius 4
  circle A37 centre (-10.1447, -51.0008) radius 4
  circle A38 centre (0, -52) radius 4
  circle A39 centre (10.1447, -51.0008) radius 4
  circle A40 centre (19.8995, -48.0417) radius 4
  circle A41 centre (28.8897, -43.2364) radius 4
  circle A42 centre (36.7696, -36.7696) radius 4
  circle A43 centre (43.2364, -28.8897) radius 4
  circle A44 centre (48.0417, -19.8995) radius 4
  circle A45 centre (51.0008, -10.1447) radius 4
  circle A46 centre (52, 0) radius 4
  circle A47 centre (51.0008, 10.1447) radius 4
  circle A48 centre (48.0417, 19.8995) radius 4
  circle A49 centre (43.2364, 28.8897) radius 4
  circle A50 centre (36.7696, 36.7696) radius 4
  circle A51 centre (28.8897, 43.2364) radius 4
  circle A52 centre (19.8995, 48.0417) radius 4
  circle A53 centre (10.1447, 51.0008) radius 4
  circle A54 centre (28.8897, 43.2364) radius 5 construction
  line L10 (0, 0) -> (26.4906, 49.3381)
  arc A55 (54.924, 10.9251) -> (10.9251, 54.924) centre (0, 0) ccw
  line L11 (0, 0) -> (35.4449, 43.355)
  line L12 (0, 0) -> (5.5933, 55.72)
  line L13 (0, 0) -> (16.1556, 53.619)
  line L14 (0, 0) -> (-16.1556, 53.619)
  line L15 (0, 0) -> (-5.5933, 55.72)
  line L16 (0, 0) -> (-35.4449, 43.355)
  line L17 (0, 0) -> (-26.4906, 49.3381)
  line L18 (0, 0) -> (-49.3381, 26.4906)
  line L19 (0, 0) -> (-43.355, 35.4449)
  line L20 (0, 0) -> (-55.72, 5.5933)
  line L21 (0, 0) -> (-53.619, 16.1556)
  line L22 (0, 0) -> (-53.619, -16.1556)
  line L23 (0, 0) -> (-55.72, -5.5933)
  line L24 (0, 0) -> (-43.355, -35.4449)
  line L25 (0, 0) -> (-49.3381, -26.4906)
  line L26 (0, 0) -> (-26.4906, -49.3381)
  line L27 (0, 0) -> (-35.4449, -43.355)
  line L28 (0, 0) -> (-5.5933, -55.72)
  line L29 (0, 0) -> (-16.1556, -53.619)
  line L30 (0, 0) -> (16.1556, -53.619)
  line L31 (0, 0) -> (5.5933, -55.72)
  line L32 (0, 0) -> (35.4449, -43.355)
  line L33 (0, 0) -> (26.4906, -49.3381)
  line L34 (0, 0) -> (49.3381, -26.4906)
  line L35 (0, 0) -> (43.355, -35.4449)
  line L36 (0, 0) -> (55.72, -5.5933)
  line L37 (0, 0) -> (53.619, -16.1556)
  line L38 (0, 0) -> (53.619, 16.1556)
  line L39 (0, 0) -> (55.72, 5.5933)
  line L40 (0, 0) -> (43.355, 35.4449)
  line L41 (0, 0) -> (49.3381, 26.4906)
  point P0 (21.756, -43.9053)
  point P1 (-3.2981, -48.8889)
  point P2 (-48.0585, -9.5594)
  point P3 (48.0585, 9.5594)
  point P4 (-46.765, 4.6944)
  point P5 (-45.0017, 13.5592)
  point P6 (-41.4087, 22.2332)
  point P7 (-36.3872, 29.7484)
  point P8 (13.5592, -45.0017)
  point P9 (4.6944, -46.765)
  point P10 (36.3872, 29.7484)
  point P11 (41.4087, 22.2332)
  point P12 (22.2332, 41.4087)
  point P13 (29.7484, 36.3872)
  point P14 (48.4591, 17.4346)
  point P15 (34.652, 38.0984)
  point P16 (17.4346, 48.4591)
  point P17 (-38.0984, 34.652)
  point P18 (-21.9376, 46.5939)
  point P19 (2.437, 51.4423)
  point P20 (-48.4591, 17.4346)
  point P21 (-51.4423, 2.437)
  point P22 (-13.5592, -45.0017)
  point P23 (-22.2332, -41.4087)
  point P24 (41.4087, -22.2332)
  dimension "d226" = 104
  dimension "d224" = 94
  dimension "d225" = 112
  dimension "d227" = 6
  dimension "d228" = 360
  dimension "d229" = 7
  dimension "d230" = 7
  dimension "d231" = 98
  dimension "d232" = 8
  dimension "d233" = 360
  dimension "d234" = 10
  dimension "d235" = 360
  constraints: 84 end point, 55 centre point, 10 coincident, 6 point on circle, 4 collinear, 4 tangent, 1 vertical alignment, 195 other
  measures "d224" diameter of A0
  measures "d225" diameter of A1
  measures "d227" diameter of A3
  measures "d229" diameter of A19
  measures "d230" diameter of A20
  measures "d231" diameter of A21
  measures "d232" diameter of A22
  measures "d234" diameter of A54
hole "Bohrung6" at (-48.0417, 19.8995, 10) at (-36.7696, 36.7696, 10) at (-19.8995, 48.0417, 10) at (36.7696, 36.7696, 10) at (48.0417, 19.8995, 10) at (52, 0, 10) direction (0, 0, 1) diameter 6 end through all
equation "\"d1\" = Aussenradius"
equation "\"d2\" = 0.5 * Innenradius + 0.5 * Aussenradius"
equation "\"d0\" = Innenradius"
equation "\"d7\" = PlateaudurchmesserObererMount"
equation "\"d8\" = PlateaudurchmesserObererMount"
equation "\"d9\" = PlateaudurchmesserObererMount"
equation "\"d10\" = PlateaudurchmesserObererMount"
equation "\"d11\" = PlateaudurchmesserObererMount"
equation "\"d12\" = Plateaudurchmesser"
equation "\"d13\" = Plateaudurchmesser"
equation "\"d14\" = Plateaudurchmesser"
equation "\"d15\" = Plateaudurchmesser"
equation "\"d16\" = Plateaudurchmesser"
equation "\"d19\" = Innenradius"
equation "\"d81\" = d95"
equation "\"d82\" = 0.5 * d94 + 0.5 * d95"
equation "\"d20\" = Aussenradius"
equation "\"d21\" = ExtrusionVerbindungselemente"
equation "\"d30\" = Innenradius"
equation "\"d31\" = Aussenradius"
equation "\"d32\" = ExtrusionVerbindungsring"
equation "\"AuslegerBreite\" = 92.1"
equation "\"d34\" = AuslegerLaenge"
equation "\"d37\" = -0.5 * d40 + 0.5 * AuslegerBreite"
equation "\"d39\" = AuslegerBreite"
equation "\"d55\" = Aussenradius"
equation "\"d35\" = AulegerDicke"
equation "\"d59\" = d73"
equation "\"d60\" = 0.5 * d72 + 0.5 * d73"
equation "\"d62\" = d74"
equation "\"d63\" = d74"
equation "\"d64\" = d74"
equation "\"d65\" = d74"
equation "\"d66\" = d74"
equation "\"d67\" = d75"
equation "\"d68\" = d75"
equation "\"d69\" = d75"
equation "\"d70\" = d75"
equation "\"d71\" = d75"
equation "\"ExtrusionVerbindungselemente\" = 10"
equation "\"ExtrusionVerbindungsring\" = 10"
equation "\"AuslegerLaenge\" = LochabstandVomZentrum - LochabstandWand"
equation "\"AulegerDicke\" = 7"
equation "\"m4\" = 4"
equation "\"LochabstandHalterungZentral\" = 19"
equation "\"LochabstandWand\" = 19"
equation "\"LochabstandHalterungAussen\" = 85"
equation "\"LochabstandVomZentrum\" = 56.49"
equation "\"d117\" = 94"
equation "\"d118\" = 112"
equation "\"d119\" = 104"
equation "\"d120\" = 5"
equation "\"d121\" = 7"
equation "\"d122\" = 94"
equation "\"d123\" = 5"
equation "\"d124\" = 10"
equation "\"d125\" = 112"
equation "\"HoehenfixierungSchaft\" = 3.2"
equation "\"StufenhoeheFuerNewport\" = 3"
equation "\"MittelpunktZuAussenseiteNewport\" = 76.2"
equation "\"NewportFusshoehe\" = 35.1"
equation "\"StufenbreiteNewport\" = 25"
equation "\"NewportSchraubenhoehe\" = 19"
equation "\"NewportSchraubenabstand\" = 12.5"
equation "\"NewportSchraubendurchmesser\" = 6.6"
equation "\"d179\" = 12"
equation "\"d208\" = 98"
equation "\"d209\" = 112"
equation "\"d210\" = 104"
equation "\"d211\" = 5"
equation "\"d212\" = 7"
equation "\"d213\" = 98"
equation "\"d214\" = 5"
equation "\"d215\" = 10"
equation "\"d216\" = 112"
equation "\"d217\" = 20"
equation "\"d236\" = 94"
equation "\"d237\" = 112"
equation "\"d238\" = 104"
equation "\"d239\" = 6"
equation "\"d240\" = 7"
equation "\"d241\" = 98"
equation "\"d242\" = 8"
equation "\"d243\" = 10"
equation "\"Aussenradius\" = 112"
equation "\"Innenradius\" = 94"
equation "\"PlateaudurchmesserObererMount\" = 12"
equation "\"Plateaudurchmesser\" = 10"
equation "\"d95\" = 112"
equation "\"d94\" = 98"
equation "\"d73\" = 112"
equation "\"d72\" = 98"
equation "\"d74\" = 12"
equation "\"d75\" = 10"
